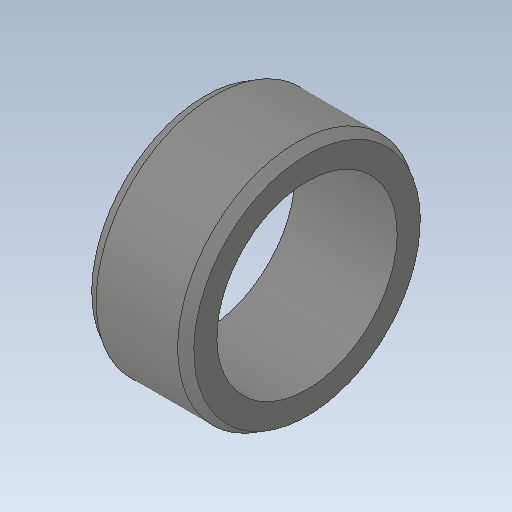
# Autodesk Inventor part: 186717 ZBH-7
Saved by Autodesk Inventor 2020 (Build 240168000, 168)
## iProperties
Created: 2023-01-29
Part Number: 186717 ZBH-7
Material: Generic
Catalog Web Link: www.cadenas.de
Description: ZBH-centring sleeve
Vendor: FESTO
Document SubType Name: Modeling
Designer: psAdmin
Manufacturer: FESTO
Mass: 0.0481442 g
Surface Area: 1.43005 cm^2
Volume: 0.0481442 cm^3
Density: 1 g/cm^3
Appearance: PSOLRGB-128-128-128
Category: PARTsolutions
Company: FESTO
PSOL_IDENT_0: {$CADENAS_DATA/23d-libs/festo/parts/z/zbh/zbh.prj},161 {VTYP=3D},{NB=186717 ZBH-7},{LINA=186717 ZBH-
PSOL_IDENT_1: 7},{NN=ZBH},{DATE=16.12.2022 17:12:13},{GEOMDATE=16.12.2022 17:12:06},{VERSION=},{LINEID=20},{WBVAR=
PSOL_IDENT_2: },{WBNUMERIC=}  {NB=186717 ZBH-7},{LINA=186717 ZBH-7},{KT=DUMMY},{TNR=186717},{TYP=ZBH-7},{INFO=2023
PSOL_IDENT_3: -12-31},{B1=3.000},{D1=7.000},{D2=5.300},{CNSMASSEXACT=0.000},{V=1},{D01=0.000},{EOLDATE=31.12.2023}
NB: 186717 ZBH-7
NN: ZBH
NT: centring sleeve
NBSYN: $TNR. $TYP.
LINA: 186717 ZBH-7
CATALOG: Festo
TNR: 186717
TYP: ZBH-7
INFO: 2023-12-31
B1: 3
D1: 7
D2: 5.3
CNSMASSEXACT: 0
SUPPLIER: FESTO
ARTICLENO: 186717 ZBH-7
BOMINFO: 186717 ZBH-7
CREATOR: CADENAS GmbH
Title: 186717 ZBH-7
Author: Cadenas PARTsolutions
Comments: centring sleeve
Autodesk Inventor part; units mm, degrees
sketch "Sketch_1" plane through (0, 0, 0) normal (0, 0, 1) x (1, 0, 0)
  line L0 (3, 0) -> (0, 0)
  line L1 (0, 2.65) -> (3, 2.65)
  line L2 (3, 2.65) -> (3, 3.3268)
  line L3 (3, 3.3268) -> (2.7, 3.5)
  line L4 (2.7, 3.5) -> (0.3, 3.5)
  line L5 (0.3, 3.5) -> (0, 3.3268)
  line L6 (0, 3.3268) -> (0, 2.65)
  constraints: 14 end point
revolve "Revolution1" add sketch "Sketch_1" angle 360 about axis through (3, 0, 0) along (-1, 0, 0)
ref_plane "anbau_XY" through (0, 0, 0) normal (1, 0, 0) x (0, 0, -1)
ref_plane "anbau_YZ" through (0, 0, 0) normal (0, 0, -1) x (0, 1, 0)
ref_plane "anbau_ZX" through (0, 0, 0) normal (0, 1, 0) x (1, 0, 0)
ref_plane "insert_XY" through (0, 0, 0) normal (1, 0, 0) x (0, 0, -1)
ref_plane "insert_YZ" through (0, 0, 0) normal (0, 0, -1) x (0, 1, 0)
ref_plane "insert_ZX" through (0, 0, 0) normal (0, 1, 0) x (1, 0, 0)
ref_plane "schraube_punkt_XY" through (3, 0, 0) normal (1, 0, 0) x (0, 0, -1)
ref_plane "schraube_punkt_YZ" through (3, 0, 0) normal (0, 0, -1) x (0, 1, 0)
ref_plane "schraube_punkt_ZX" through (3, 0, 0) normal (0, 1, 0) x (1, 0, 0)
body "Solid1"
